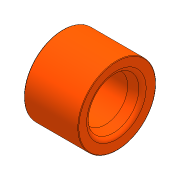
# Autodesk Inventor part: Kegel_urethane
Saved by Autodesk Inventor 2017 (Build 210142000, 142)
## iProperties
Created: 2018-01-15
Part Number: Kegel_urethane
Material: Rubber, Silicone
Document SubType Name: Modeling
Designer: Tobias
Density: 1.25 g/cm^3
Appearance: Rubber - Black(2)
Mass: 215.384 g
Surface Area: 275.965 cm^2
Volume: 172.308 cm^3
Author: Tobias
Autodesk Inventor part; units mm, degrees
ref_plane "YZ Plane" through (0, 0, 0) normal (1, 0, 0) x (0, 1, 0)
ref_plane "XZ Plane" through (0, 0, 0) normal (0, 1, 0) x (-1, 0, 0)
ref_plane "XY Plane" through (0, 0, 0) normal (0, 0, 1) x (1, 0, 0)
sketch "Sketch1" plane through (0, 0, 0) normal (0, 0, 1) x (1, 0, 0)
  line L0 (-35.8, 0) -> (42.6, 0) projected
  line L1 (30.3064, 27.5) -> (19, 23.25)
  line L2 (19, 23.25) -> (-19, 23.25)
  line L3 (-24.1407, 34.75) -> (-23.2, 34.75)
  line L4 (-23.2, 34.75) -> (-23.2, 31.5)
  line L5 (-23.2, 31.5) -> (-19, 31.5)
  line L6 (-19, 31.5) -> (-19, 23.25)
  line L7 (31.4, 40) -> (30.3064, 27.5)
  line L8 (-24.6, 40) -> (-24.1407, 34.75)
  line L9 (-24.6, 40) -> (31.4, 40)
  line L10 (0, 48) -> (0, -8) projected
  point P0 (0, 0)
  dimension "d27" = 46.5
  dimension "d29" = 69.5
  dimension "d31" = 63
  dimension "d35" = 55
  dimension "d39" = 80
  dimension "d40" = 1.4
  dimension "d42" = 5.6
  dimension "d44" = 19
  dimension "d45" = 19
  dimension "d46" = 56
  dimension "d47" = 5
  dimension "d48" = 5
  dimension "d49" = 12.5
  constraints: 18 end point, 3 perpendicular, 2 horizontal
  measures "d27" diameter of L2 L0
  measures "d29" diameter of L3 L0
  measures "d31" diameter of L5 L0
  measures "d35" diameter of L1.start L0
  measures "d39" diameter of L9 L0
  measures "d40" distance from line of L8.start L4
  measures "d42" distance from line of L6 L8.start
  measures "d44" distance between parallel lines of L10 L6
  measures "d45" distance from line of L10 L1.end
  measures "d46" distance of L8.start L7.start
  measures "d47" angle of L10 L8
  measures "d48" angle of L10 L7
  measures "d49" distance from line of L1.start L9
revolve "Revolution1" add sketch "Sketch1" angle 360 about axis through (0, 0, 0) along (1, 0, 0)
fillet "Fillet8" radius 7 1 edges at (-19, -31.5, 0)
fillet "Fillet9" radius 7 1 edges at (-23.2, -31.5, 0)
fillet "Fillet10" radius 6 1 edges at (-23.2, -34.75, 0)
fillet "Fillet11" radius 5 1 edges at (30.3064, -27.5, 0)
fillet "Fillet12" radius 0.5 2 edges at (31.4, -40, 0) (-24.6, -40, 0)
body "Solid1"
